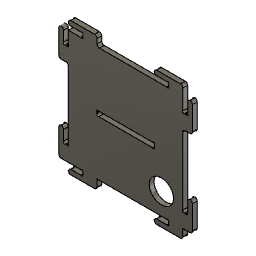
Side_HeatGun_Cut1 (Autodesk Fusion 360 design; units mm, degrees)
Autodesk Fusion 360 part; units mm, degrees
sketch "Sketch1" plane through (0, 0, 0) normal (0, 0, 1) x (1, 0, 0)
  line L0 (0, 0) -> (304.8, 0)
  line L1 (304.8, 0) -> (304.8, -304.8)
  line L2 (304.8, -304.8) -> (0, -304.8)
  line L3 (0, -304.8) -> (0, 0)
  line L4 (304.8, 0) -> (304.8, 25.4)
  line L5 (304.8, -304.8) -> (304.8, -330.2)
  line L6 (0, 0) -> (76.2, 0) construction
  line L7 (0, -304.8) -> (76.2, -304.8) construction
  line L8 (76.2, -304.8) -> (76.2, -330.2)
  line L9 (304.8, -330.2) -> (228.6, -330.2)
  line L10 (76.2, -330.2) -> (0, -330.2)
  line L11 (0, -330.2) -> (0, -317.5)
  line L12 (0, -317.5) -> (38.1, -317.5)
  line L13 (38.1, -317.5) -> (38.1, -304.8)
  line L14 (228.6, -330.2) -> (228.6, -317.5)
  line L15 (228.6, -317.5) -> (266.7, -317.5)
  line L16 (266.7, -317.5) -> (266.7, -304.8)
  line L17 (304.8, 25.4) -> (228.6, 25.4)
  line L18 (228.6, 25.4) -> (228.6, 12.7)
  line L19 (228.6, 12.7) -> (266.7, 12.7)
  line L20 (266.7, 12.7) -> (266.7, 0)
  line L21 (76.2, 0) -> (76.2, 25.4)
  line L22 (76.2, 25.4) -> (0, 25.4)
  line L23 (0, 25.4) -> (0, 12.7)
  line L24 (0, 12.7) -> (38.1, 12.7)
  line L25 (38.1, 12.7) -> (38.1, 0)
  line L26 (152.4, 0) -> (152.4, -152.4) construction
  line L27 (228.6, -158.75) -> (76.2, -158.75)
  line L28 (76.2, -158.75) -> (76.2, -146.05)
  line L29 (76.2, -146.05) -> (228.6, -146.05)
  line L30 (228.6, -146.05) -> (228.6, -158.75)
  line L31 (228.6, -158.75) -> (76.2, -146.05) construction
  line L32 (76.2, -158.75) -> (228.6, -146.05) construction
  line L33 (0, 0) -> (0, -76.2) construction
  line L34 (0, -76.2) -> (-25.4, -76.2)
  line L35 (-25.4, -76.2) -> (-25.4, 0)
  line L36 (-25.4, 0) -> (-12.7, 0)
  line L37 (-12.7, 0) -> (-12.7, -38.1)
  line L38 (-12.7, -38.1) -> (0, -38.1)
  line L39 (0, -304.8) -> (-25.4, -304.8)
  line L40 (-25.4, -304.8) -> (-25.4, -228.6)
  line L41 (-25.4, -228.6) -> (-12.7, -228.6)
  line L42 (-12.7, -228.6) -> (-12.7, -266.7)
  line L43 (-12.7, -266.7) -> (0, -266.7)
  line L44 (304.8, -304.8) -> (330.2, -304.8)
  line L45 (330.2, -304.8) -> (330.2, -228.6)
  line L46 (330.2, -228.6) -> (317.5, -228.6)
  line L47 (317.5, -228.6) -> (317.5, -266.7)
  line L48 (317.5, -266.7) -> (304.8, -266.7)
  line L49 (304.8, 0) -> (304.8, -76.2) construction
  line L50 (304.8, -76.2) -> (330.2, -76.2)
  line L51 (330.2, -76.2) -> (330.2, 0)
  line L52 (330.2, 0) -> (317.5, 0)
  line L53 (317.5, 0) -> (317.5, -38.1)
  line L54 (317.5, -38.1) -> (304.8, -38.1)
  point P0 (152.4, -152.4)
  dimension "d1" = 304.8
  dimension "d2" = 304.8
  dimension "d3" = 25.4
  dimension "d4" = 25.4
  dimension "d5" = 76.2
  dimension "d6" = 76.2
  dimension "d7" = 25.4
  dimension "d8" = 76.2
  dimension "d9" = 12.7
  dimension "d10" = 76.2
  dimension "d11" = 38.1
  dimension "d12" = 25.4
  dimension "d13" = 38.1
  dimension "d14" = 152.4
  dimension "d15" = 152.4
  dimension "d16" = 12.7
  dimension "d17" = 76.2
  dimension "d18" = 25.4
  dimension "d19" = 76.2
  dimension "d20" = 12.7
  dimension "d21" = 38.1
  dimension "d22" = 76.2
  dimension "d23" = 38.1
  dimension "d24" = 76.2
  constraint horizontal L0
  constraint vertical L1
  constraint horizontal L2
  constraint vertical L3
  constraint coincident L0.start L3.end
  constraint perpendicular L0 L4
  constraint perpendicular L2 L5
  constraint perpendicular L3 L6
  constraint perpendicular L3 L7
  constraint perpendicular L2 L8
  constraint perpendicular L5 L9
  constraint perpendicular L8 L10
  constraint perpendicular L10 L11
  constraint perpendicular L11 L12
  constraint midpoint L7 L13.end
  constraint perpendicular L9 L14
  constraint perpendicular L14 L15
  constraint coincident L2 L16.end
  constraint perpendicular L2 L16
  constraint perpendicular L4 L17
  constraint perpendicular L17 L18
  constraint perpendicular L4 L19
  constraint coincident L0 L20.end
  constraint perpendicular L0 L20
  constraint perpendicular L0 L21
  constraint perpendicular L21 L22
  constraint perpendicular L22 L23
  constraint perpendicular L21 L24
  constraint midpoint L6 L25.end
  constraint perpendicular L6 L25
  constraint midpoint L0 L26.start
  constraint perpendicular L2 L26
  constraint horizontal L27
  constraint perpendicular L27 L28
  constraint parallel L27 L29
  constraint parallel L28 L30
  constraint coincident L31 P0
  constraint coincident L32 P0
  constraint coincident P0 L26.end
  constraint perpendicular L0 L33
  constraint perpendicular L3 L34
  constraint perpendicular L34 L35
  constraint perpendicular L35 L36
  constraint perpendicular L36 L37
  constraint midpoint L33 L38.end
  constraint perpendicular L3 L39
  constraint perpendicular L39 L40
  constraint perpendicular L40 L41
  constraint perpendicular L41 L42
  constraint coincident L3 L43.end
  constraint perpendicular L3 L43
  constraint perpendicular L5 L44
  constraint perpendicular L2 L45
  constraint perpendicular L5 L46
  constraint perpendicular L46 L47
  constraint coincident L1 L48.end
  constraint perpendicular L1 L48
  constraint perpendicular L0 L49
  constraint perpendicular L1 L50
  constraint perpendicular L50 L51
  constraint perpendicular L1 L52
  constraint perpendicular L50 L53
  constraint midpoint L49 L54.end
  constraint perpendicular L49 L54
  measures "d1" distance of L0.start L0.end
  measures "d2" distance of L0.start L2.end
  measures "d3" distance of L0.end L4.end
  measures "d4" distance of L1.end L5.end
  measures "d5" distance of L0.start L6.end
  measures "d6" distance of L2.end L7.end
  measures "d7" distance of L7.end L8.end
  measures "d8" distance of L5.end L9.end
  measures "d9" distance of L9.end L14.end
  measures "d10" distance of L4.end L17.end
  measures "d11" distance of L18.end L19.end
  measures "d12" distance of L6.end L21.end
  measures "d13" distance of L23.end L24.end
  measures "d14" distance of L26.start P0
  measures "d15" distance of L28.end L29.end
  measures "d16" distance of L27.end L28.end
  measures "d17" distance of L0.start L33.end
  measures "d18" distance of L33.end L34.end
  measures "d19" distance of L34.end L35.end
  measures "d20" distance of L35.end L36.end
  measures "d21" distance of L36.end L37.end
  measures "d22" distance of L39.end L40.end
  measures "d23" distance of L41.end L42.end
  measures "d24" distance of L0.end L49.end
extrude "Extrude1" add sketch "Sketch1" along normal blind 12.7 makes body 1
fillet "Fillet1" radius 6.35 27 edges at (-25.4, 0, 6.35) (-12.7, 0, 6.35) (-25.4, -76.2, 6.35) (0, -76.2, 6.35) (0, 25.4, 6.35) (0, 12.7, 6.35) (76.2, 25.4, 6.35) (76.2, 0, 6.35) (228.6, 25.4, 6.35) (228.6, 12.7, 6.35) (304.8, 25.4, 6.35) (317.5, 0, 6.35) (330.2, 0, 6.35) (330.2, -76.2, 6.35) (304.8, -76.2, 6.35) (330.2, -228.6, 6.35) (317.5, -228.6, 6.35) (330.2, -304.8, 6.35) (304.8, -330.2, 6.35) (228.6, -317.5, 6.35) (228.6, -330.2, 6.35) (0, -317.5, 6.35) (0, -330.2, 6.35) (76.2, -330.2, 6.35) (-25.4, -304.8, 6.35) (-25.4, -228.6, 6.35) (-12.7, -228.6, 6.35) on bodies 1
sketch "Sketch2" plane through (0, 0, 12.7) normal (0, 0, 1) x (1, 0, 0)
  arc A0 (-12.7, -234.95) -> (-19.05, -228.6) centre (-19.05, -234.95) ccw
  arc A1 (-19.05, -228.6) -> (-25.4, -234.95) centre (-19.05, -234.95) ccw
  line L0 (-25.4, -234.95) -> (-25.4, -298.45)
  arc A2 (-25.4, -298.45) -> (-19.05, -304.8) centre (-19.05, -298.45) ccw
  line L1 (-19.05, -304.8) -> (38.1, -304.8)
  line L2 (38.1, -304.8) -> (38.1, -317.5)
  line L3 (38.1, -317.5) -> (6.35, -317.5)
  arc A3 (6.35, -317.5) -> (0, -323.85) centre (6.35, -323.85) ccw
  arc A4 (0, -323.85) -> (6.35, -330.2) centre (6.35, -323.85) ccw
  line L4 (6.35, -330.2) -> (69.85, -330.2)
  arc A5 (69.85, -330.2) -> (76.2, -323.85) centre (69.85, -323.85) ccw
  line L5 (76.2, -323.85) -> (76.2, -304.8)
  line L6 (76.2, -304.8) -> (266.7, -304.8)
  line L7 (266.7, -304.8) -> (266.7, -317.5)
  line L8 (266.7, -317.5) -> (234.95, -317.5)
  arc A6 (234.95, -317.5) -> (234.95, -330.2) centre (234.95, -323.85) ccw
  line L9 (234.95, -330.2) -> (298.45, -330.2)
  arc A7 (298.45, -330.2) -> (304.8, -323.85) centre (298.45, -323.85) ccw
  line L10 (304.8, -323.85) -> (304.8, -304.8)
  line L11 (304.8, -304.8) -> (323.85, -304.8)
  arc A8 (323.85, -304.8) -> (330.2, -298.45) centre (323.85, -298.45) ccw
  line L12 (330.2, -298.45) -> (330.2, -234.95)
  arc A9 (330.2, -234.95) -> (323.85, -228.6) centre (323.85, -234.95) ccw
  arc A10 (323.85, -228.6) -> (317.5, -234.95) centre (323.85, -234.95) ccw
  line L13 (317.5, -234.95) -> (317.5, -266.7)
  line L14 (317.5, -266.7) -> (304.8, -266.7)
  line L15 (304.8, -266.7) -> (304.8, -82.55)
  arc A11 (311.15, -76.2) -> (304.8, -82.55) centre (311.15, -82.55) ccw
  line L16 (311.15, -76.2) -> (323.85, -76.2)
  arc A12 (323.85, -76.2) -> (330.2, -69.85) centre (323.85, -69.85) ccw
  line L17 (330.2, -69.85) -> (330.2, -6.35)
  arc A13 (330.2, -6.35) -> (323.85, 0) centre (323.85, -6.35) ccw
  arc A14 (323.85, 0) -> (317.5, -6.35) centre (323.85, -6.35) ccw
  line L18 (317.5, -6.35) -> (317.5, -38.1)
  line L19 (317.5, -38.1) -> (304.8, -38.1)
  line L20 (304.8, -38.1) -> (304.8, 19.05)
  arc A15 (304.8, 19.05) -> (298.45, 25.4) centre (298.45, 19.05) ccw
  line L21 (298.45, 25.4) -> (234.95, 25.4)
  arc A16 (234.95, 25.4) -> (228.6, 19.05) centre (234.95, 19.05) ccw
  arc A17 (228.6, 19.05) -> (234.95, 12.7) centre (234.95, 19.05) ccw
  line L22 (234.95, 12.7) -> (266.7, 12.7)
  line L23 (266.7, 12.7) -> (266.7, 0)
  line L24 (266.7, 0) -> (82.55, 0)
  arc A18 (76.2, 6.35) -> (82.55, 0) centre (82.55, 6.35) ccw
  line L25 (76.2, 6.35) -> (76.2, 19.05)
  arc A19 (76.2, 19.05) -> (69.85, 25.4) centre (69.85, 19.05) ccw
  line L26 (69.85, 25.4) -> (6.35, 25.4)
  arc A20 (6.35, 25.4) -> (6.35, 12.7) centre (6.35, 19.05) ccw
  line L27 (6.35, 12.7) -> (38.1, 12.7)
  line L28 (38.1, 12.7) -> (38.1, 0)
  line L29 (38.1, 0) -> (0, 0)
  line L30 (0, 0) -> (0, -38.1)
  line L31 (0, -38.1) -> (-12.7, -38.1)
  line L32 (-12.7, -38.1) -> (-12.7, -6.35)
  arc A21 (-12.7, -6.35) -> (-25.4, -6.35) centre (-19.05, -6.35) ccw
  line L33 (-25.4, -6.35) -> (-25.4, -69.85)
  arc A22 (-25.4, -69.85) -> (-19.05, -76.2) centre (-19.05, -69.85) ccw
  line L34 (-19.05, -76.2) -> (-6.35, -76.2)
  arc A23 (0, -82.55) -> (-6.35, -76.2) centre (-6.35, -82.55) ccw
  line L35 (0, -82.55) -> (0, -266.7)
  line L36 (0, -266.7) -> (-12.7, -266.7)
  line L37 (-12.7, -266.7) -> (-12.7, -234.95)
  line L38 (76.2, -146.05) -> (228.6, -146.05)
  line L39 (228.6, -146.05) -> (228.6, -158.75)
  line L40 (228.6, -158.75) -> (76.2, -158.75)
  line L41 (76.2, -158.75) -> (76.2, -146.05)
copy_body "Body->Comp1" bodies 1 removing the originals makes body 2 in component "Component"
sketch "Sketch3" plane through (0, 0, 12.7) normal (0, 0, 1) x (1, 0, 0)
  arc A0 (-12.7, -234.95) -> (-19.05, -228.6) centre (-19.05, -234.95) ccw
  arc A1 (-19.05, -228.6) -> (-25.4, -234.95) centre (-19.05, -234.95) ccw
  line L0 (-25.4, -234.95) -> (-25.4, -298.45)
  arc A2 (-25.4, -298.45) -> (-19.05, -304.8) centre (-19.05, -298.45) ccw
  line L1 (-19.05, -304.8) -> (38.1, -304.8)
  line L2 (38.1, -304.8) -> (38.1, -317.5)
  line L3 (38.1, -317.5) -> (6.35, -317.5)
  arc A3 (6.35, -317.5) -> (0, -323.85) centre (6.35, -323.85) ccw
  arc A4 (0, -323.85) -> (6.35, -330.2) centre (6.35, -323.85) ccw
  line L4 (6.35, -330.2) -> (69.85, -330.2)
  arc A5 (69.85, -330.2) -> (76.2, -323.85) centre (69.85, -323.85) ccw
  line L5 (76.2, -323.85) -> (76.2, -304.8)
  line L6 (76.2, -304.8) -> (266.7, -304.8)
  line L7 (266.7, -304.8) -> (266.7, -317.5)
  line L8 (266.7, -317.5) -> (234.95, -317.5)
  arc A6 (234.95, -317.5) -> (234.95, -330.2) centre (234.95, -323.85) ccw
  line L9 (234.95, -330.2) -> (298.45, -330.2)
  arc A7 (298.45, -330.2) -> (304.8, -323.85) centre (298.45, -323.85) ccw
  line L10 (304.8, -323.85) -> (304.8, -304.8)
  line L11 (304.8, -304.8) -> (323.85, -304.8)
  arc A8 (323.85, -304.8) -> (330.2, -298.45) centre (323.85, -298.45) ccw
  line L12 (330.2, -298.45) -> (330.2, -234.95)
  arc A9 (330.2, -234.95) -> (323.85, -228.6) centre (323.85, -234.95) ccw
  arc A10 (323.85, -228.6) -> (317.5, -234.95) centre (323.85, -234.95) ccw
  line L13 (317.5, -234.95) -> (317.5, -266.7)
  line L14 (317.5, -266.7) -> (304.8, -266.7)
  line L15 (304.8, -266.7) -> (304.8, -82.55)
  arc A11 (311.15, -76.2) -> (304.8, -82.55) centre (311.15, -82.55) ccw
  line L16 (311.15, -76.2) -> (323.85, -76.2)
  arc A12 (323.85, -76.2) -> (330.2, -69.85) centre (323.85, -69.85) ccw
  line L17 (330.2, -69.85) -> (330.2, -6.35)
  arc A13 (330.2, -6.35) -> (323.85, 0) centre (323.85, -6.35) ccw
  arc A14 (323.85, 0) -> (317.5, -6.35) centre (323.85, -6.35) ccw
  line L18 (317.5, -6.35) -> (317.5, -38.1)
  line L19 (317.5, -38.1) -> (304.8, -38.1)
  line L20 (304.8, -38.1) -> (304.8, 19.05)
  arc A15 (304.8, 19.05) -> (298.45, 25.4) centre (298.45, 19.05) ccw
  line L21 (298.45, 25.4) -> (234.95, 25.4)
  arc A16 (234.95, 25.4) -> (228.6, 19.05) centre (234.95, 19.05) ccw
  arc A17 (228.6, 19.05) -> (234.95, 12.7) centre (234.95, 19.05) ccw
  line L22 (234.95, 12.7) -> (266.7, 12.7)
  line L23 (266.7, 12.7) -> (266.7, 0)
  line L24 (266.7, 0) -> (82.55, 0)
  arc A18 (76.2, 6.35) -> (82.55, 0) centre (82.55, 6.35) ccw
  line L25 (76.2, 6.35) -> (76.2, 19.05)
  arc A19 (76.2, 19.05) -> (69.85, 25.4) centre (69.85, 19.05) ccw
  line L26 (69.85, 25.4) -> (6.35, 25.4)
  arc A20 (6.35, 25.4) -> (6.35, 12.7) centre (6.35, 19.05) ccw
  line L27 (6.35, 12.7) -> (38.1, 12.7)
  line L28 (38.1, 12.7) -> (38.1, 0)
  line L29 (38.1, 0) -> (0, 0)
  line L30 (0, 0) -> (0, -38.1)
  line L31 (0, -38.1) -> (-12.7, -38.1)
  line L32 (-12.7, -38.1) -> (-12.7, -6.35)
  arc A21 (-12.7, -6.35) -> (-25.4, -6.35) centre (-19.05, -6.35) ccw
  line L33 (-25.4, -6.35) -> (-25.4, -69.85)
  arc A22 (-25.4, -69.85) -> (-19.05, -76.2) centre (-19.05, -69.85) ccw
  line L34 (-19.05, -76.2) -> (-6.35, -76.2)
  arc A23 (0, -82.55) -> (-6.35, -76.2) centre (-6.35, -82.55) ccw
  line L35 (0, -82.55) -> (0, -266.7)
  line L36 (0, -266.7) -> (-12.7, -266.7)
  line L37 (-12.7, -266.7) -> (-12.7, -234.95)
  line L38 (76.2, -146.05) -> (228.6, -146.05)
  line L39 (228.6, -146.05) -> (228.6, -158.75)
  line L40 (228.6, -158.75) -> (76.2, -158.75)
  line L41 (76.2, -158.75) -> (76.2, -146.05)
  line L42 (304.8, -304.8) -> (247.65, -304.8) construction
  line L43 (247.65, -304.8) -> (247.65, -247.65) construction
  ellipse E0 centre (247.65, -247.65) end of major axis (247.65, -216.535) minor radius 32.385
  line L44 (247.65, -278.765) -> (247.65, -216.535)
  line L45 (280.035, -247.65) -> (215.265, -247.65)
  dimension "d29" = 57.15
  dimension "d30" = 57.15
  dimension "d32" = 62.23
  dimension "d33" = 64.77
  constraint coincident L10.end L11.start
  constraint perpendicular L7 L42
  constraint perpendicular L6 L43
  constraint coincident L43.end E0.centre
  constraint parallel L43 L44
  constraint coincident E0 L44.start
  constraint coincident E0 L44.end
  constraint coincident E0 L45.start
  constraint coincident E0 L45.end
  measures "d29" distance of L10.end L42.end
  measures "d30" distance of L42.end L43.end
  measures "d32" distance of E0
extrude "Extrude1'" cut sketch "Sketch3" against normal up to surface (12.7 mm away) contours E0 L44 L45 | E0 L44 L45 | E0 L44 L45 | E0 L44 L45 bodies 2 in component "Component"
ref_plane "WorkPlane1" through (38.1, 12.7, 0) normal (0, 0, 1) x (1, 0, 0)
sketch "Sketch4" plane through (38.1, 12.7, 0) normal (0, 0, 1) x (1, 0, 0)
  line L0 (-31.75, 0) -> (0, 0) construction
  line L1 (0, 0) -> (0, -12.7) construction
  line L2 (0, 0) -> (-2.2451, -2.2451) construction
  circle A0 centre (-2.2451, -2.2451) radius 3.175
  dimension "d37" = 3.175
  constraint coincident L0.end L1.start
  constraint coincident L0.end A0
  measures "d37" distance of L0.end L2.end
sweep "Sweep1" cut kept parallel profiles "Sketch4" along 1 edges at (38.1, 12.7, 6.35) section 1 on bodies 2 bodies 2 in component "Component"
ref_plane "WorkPlane2" through (38.1, 0, 0) normal (0, 0, 1) x (1, 0, 0)
sketch "Sketch5" plane through (38.1, 0, 0) normal (0, 0, 1) x (1, 0, 0)
  line L0 (0, 8.2099) -> (0, 0) construction
  line L1 (-38.1, 0) -> (0, 0) construction
  line L2 (0, 0) -> (-2.2451, 2.2451) construction
  circle A0 centre (-2.2451, 2.2451) radius 3.175
  dimension "d45" = 3.175
  constraint coincident L0.end L1.end
  constraint coincident L0.end A0
  measures "d45" distance of L0.end L2.end
sweep "Sweep2" cut kept parallel profiles "Sketch5" along 1 edges at (38.1, 0, 6.35) section 1 on bodies 2 bodies 2 in component "Component"
ref_plane "WorkPlane3" through (0, -38.1, 0) normal (0, 0, 1) x (1, 0, 0)
sketch "Sketch6" plane through (0, -38.1, 0) normal (0, 0, 1) x (1, 0, 0)
  line L0 (0, 0) -> (0, 38.1) construction
  line L1 (-12.7, 0) -> (0, 0) construction
  line L2 (0, 0) -> (-2.2451, 2.2451) construction
  circle A0 centre (-2.2451, 2.2451) radius 3.175
  dimension "d53" = 3.175
  constraint coincident L0.start L1.end
  constraint coincident L0.start A0
  measures "d53" distance of L0.start L2.end
sweep "Sweep3" cut kept parallel profiles "Sketch6" along 1 edges at (0, -38.1, 6.35) section 1 on bodies 2 bodies 2 in component "Component"
ref_plane "WorkPlane4" through (-12.7, -38.1, 0) normal (0, 0, 1) x (1, 0, 0)
sketch "Sketch7" plane through (-12.7, -38.1, 0) normal (0, 0, 1) x (1, 0, 0)
  line L0 (0, 0) -> (8.2099, 0) construction
  line L1 (0, 31.75) -> (0, 0) construction
  line L2 (0, 0) -> (2.2451, 2.2451) construction
  circle A0 centre (2.2451, 2.2451) radius 3.175
  dimension "d61" = 3.175
  constraint coincident L0.start L1.end
  constraint coincident L0.start A0
  measures "d61" distance of L0.start L2.end
sweep "Sweep4" cut kept parallel profiles "Sketch7" along 1 edges at (-12.7, -38.1, 6.35) section 1 on bodies 2 bodies 2 in component "Component"
ref_plane "WorkPlane5" through (304.8, -38.1, 0) normal (0, 0, 1) x (1, 0, 0)
sketch "Sketch8" plane through (304.8, -38.1, 0) normal (0, 0, 1) x (1, 0, 0)
  line L0 (12.7, 0) -> (0, 0) construction
  line L1 (0, 57.15) -> (0, 0) construction
  line L2 (0, 0) -> (2.2451, 2.2451) construction
  circle A0 centre (2.2451, 2.2451) radius 3.175
  dimension "d69" = 3.175
  constraint coincident L0.end L1.end
  constraint coincident L0.end A0
  measures "d69" distance of L0.end L2.end
sweep "Sweep5" cut kept parallel profiles "Sketch8" along 1 edges at (304.8, -38.1, 6.35) section 1 on bodies 2 bodies 2 in component "Component"
ref_plane "WorkPlane6" through (317.5, -38.1, 0) normal (0, 0, 1) x (1, 0, 0)
sketch "Sketch9" plane through (317.5, -38.1, 0) normal (0, 0, 1) x (1, 0, 0)
  line L0 (0, 31.75) -> (0, 0) construction
  line L1 (0, 0) -> (-8.2099, 0) construction
  line L2 (0, 0) -> (-2.2451, 2.2451) construction
  circle A0 centre (-2.2451, 2.2451) radius 3.175
  dimension "d77" = 3.175
  constraint coincident L0.end L1.start
  constraint coincident L0.end A0
  measures "d77" distance of L0.end L2.end
sweep "Sweep6" cut kept parallel profiles "Sketch9" along 1 edges at (317.5, -38.1, 6.35) section 1 on bodies 2 bodies 2 in component "Component"
ref_plane "WorkPlane7" through (266.7, 12.7, 0) normal (0, 0, 1) x (1, 0, 0)
sketch "Sketch10" plane through (266.7, 12.7, 0) normal (0, 0, 1) x (1, 0, 0)
  line L0 (-31.75, 0) -> (0, 0) construction
  line L1 (0, 0) -> (0, -12.7) construction
  line L2 (0, 0) -> (-2.2451, -2.2451) construction
  circle A0 centre (-2.2451, -2.2451) radius 3.175
  dimension "d85" = 3.175
  constraint coincident L0.end L1.start
  constraint coincident L0.end A0
  measures "d85" distance of L0.end L2.end
sweep "Sweep7" cut kept parallel profiles "Sketch10" along 1 edges at (266.7, 12.7, 6.35) section 1 on bodies 2 bodies 2 in component "Component"
ref_plane "WorkPlane8" through (266.7, 0, 0) normal (0, 0, 1) x (1, 0, 0)
sketch "Sketch11" plane through (266.7, 0, 0) normal (0, 0, 1) x (1, 0, 0)
  line L0 (0, 8.2099) -> (0, 0) construction
  line L1 (-184.15, 0) -> (0, 0) construction
  line L2 (0, 0) -> (-2.2451, 2.2451) construction
  circle A0 centre (-2.2451, 2.2451) radius 3.175
  dimension "d93" = 3.175
  constraint coincident L0.end L1.end
  constraint coincident L0.end A0
  measures "d93" distance of L0.end L2.end
sweep "Sweep8" cut kept parallel profiles "Sketch11" along 1 edges at (266.7, 0, 6.35) section 1 on bodies 2 bodies 2 in component "Component"
ref_plane "WorkPlane9" through (317.5, -266.7, 0) normal (0, 0, 1) x (1, 0, 0)
sketch "Sketch12" plane through (317.5, -266.7, 0) normal (0, 0, 1) x (1, 0, 0)
  line L0 (0, 31.75) -> (0, 0) construction
  line L1 (0, 0) -> (-12.7, 0) construction
  line L2 (0, 0) -> (-2.2451, 2.2451) construction
  circle A0 centre (-2.2451, 2.2451) radius 3.175
  dimension "d101" = 3.175
  constraint coincident L0.end L1.start
  constraint coincident L0.end A0
  measures "d101" distance of L0.end L2.end
sweep "Sweep9" cut kept parallel profiles "Sketch12" along 1 edges at (317.5, -266.7, 6.35) section 1 on bodies 2 bodies 2 in component "Component"
ref_plane "WorkPlane10" through (304.8, -266.7, 0) normal (0, 0, 1) x (1, 0, 0)
sketch "Sketch13" plane through (304.8, -266.7, 0) normal (0, 0, 1) x (1, 0, 0)
  line L0 (8.2099, 0) -> (0, 0) construction
  line L1 (0, 184.15) -> (0, 0) construction
  line L2 (0, 0) -> (2.2451, 2.2451) construction
  circle A0 centre (2.2451, 2.2451) radius 3.175
  dimension "d109" = 3.175
  constraint coincident L0.end L1.end
  constraint coincident L0.end A0
  measures "d109" distance of L0.end L2.end
sweep "Sweep10" cut kept parallel profiles "Sketch13" along 1 edges at (304.8, -266.7, 6.35) section 1 on bodies 2 bodies 2 in component "Component"
ref_plane "WorkPlane11" through (266.7, -304.8, 0) normal (0, 0, 1) x (1, 0, 0)
sketch "Sketch14" plane through (266.7, -304.8, 0) normal (0, 0, 1) x (1, 0, 0)
  line L0 (0, 0) -> (-190.5, 0) construction
  line L1 (0, -12.7) -> (0, 0) construction
  line L2 (0, 0) -> (-2.2451, -2.2451) construction
  circle A0 centre (-2.2451, -2.2451) radius 3.175
  dimension "d117" = 3.175
  constraint coincident L0.start L1.end
  constraint coincident L0.start A0
  measures "d117" distance of L0.start L2.end
sweep "Sweep11" cut kept parallel profiles "Sketch14" along 1 edges at (266.7, -304.8, 6.35) section 1 on bodies 2 bodies 2 in component "Component"
ref_plane "WorkPlane12" through (266.7, -317.5, 0) normal (0, 0, 1) x (1, 0, 0)
sketch "Sketch15" plane through (266.7, -317.5, 0) normal (0, 0, 1) x (1, 0, 0)
  line L0 (0, 0) -> (0, 8.2099) construction
  line L1 (-31.75, 0) -> (0, 0) construction
  line L2 (0, 0) -> (-2.2451, 2.2451) construction
  circle A0 centre (-2.2451, 2.2451) radius 3.175
  dimension "d125" = 3.175
  constraint coincident L0.start L1.end
  constraint coincident L0.start A0
  measures "d125" distance of L0.start L2.end
sweep "Sweep12" cut kept parallel profiles "Sketch15" along 1 edges at (266.7, -317.5, 6.35) section 1 on bodies 2 bodies 2 in component "Component"
ref_plane "WorkPlane13" through (228.6, -158.75, 0) normal (0, 0, 1) x (1, 0, 0)
sketch "Sketch16" plane through (228.6, -158.75, 0) normal (0, 0, 1) x (1, 0, 0)
  line L0 (0, 12.7) -> (0, 0) construction
  line L1 (0, 0) -> (-152.4, 0) construction
  line L2 (0, 0) -> (-2.2451, 2.2451) construction
  circle A0 centre (-2.2451, 2.2451) radius 3.175
  dimension "d133" = 3.175
  constraint coincident L0.end L1.start
  constraint coincident L0.end A0
  measures "d133" distance of L0.end L2.end
sweep "Sweep13" cut kept parallel profiles "Sketch16" along 1 edges at (228.6, -158.75, 6.35) section 1 on bodies 2 bodies 2 in component "Component"
ref_plane "WorkPlane14" through (76.2, -158.75, 0) normal (0, 0, 1) x (1, 0, 0)
sketch "Sketch17" plane through (76.2, -158.75, 0) normal (0, 0, 1) x (1, 0, 0)
  line L0 (147.9099, 0) -> (0, 0) construction
  line L1 (0, 0) -> (0, 12.7) construction
  line L2 (0, 0) -> (2.2451, 2.2451) construction
  circle A0 centre (2.2451, 2.2451) radius 3.175
  dimension "d141" = 3.175
  constraint coincident L0.end L1.start
  constraint coincident L0.end A0
  measures "d141" distance of L0.end L2.end
sweep "Sweep14" cut kept parallel profiles "Sketch17" along 1 edges at (76.2, -158.75, 6.35) section 1 on bodies 2 bodies 2 in component "Component"
ref_plane "WorkPlane15" through (76.2, -146.05, 0) normal (0, 0, 1) x (1, 0, 0)
sketch "Sketch18" plane through (76.2, -146.05, 0) normal (0, 0, 1) x (1, 0, 0)
  line L0 (0, 0) -> (152.4, 0) construction
  line L1 (0, -8.2099) -> (0, 0) construction
  line L2 (0, 0) -> (2.2451, -2.2451) construction
  circle A0 centre (2.2451, -2.2451) radius 3.175
  dimension "d149" = 3.175
  constraint coincident L0.start L1.end
  constraint coincident L0.start A0
  measures "d149" distance of L0.start L2.end
sweep "Sweep15" cut kept parallel profiles "Sketch18" along 1 edges at (76.2, -146.05, 6.35) section 1 on bodies 2 bodies 2 in component "Component"
ref_plane "WorkPlane16" through (228.6, -146.05, 0) normal (0, 0, 1) x (1, 0, 0)
sketch "Sketch19" plane through (228.6, -146.05, 0) normal (0, 0, 1) x (1, 0, 0)
  line L0 (-147.9099, 0) -> (0, 0) construction
  line L1 (0, 0) -> (0, -8.2099) construction
  line L2 (0, 0) -> (-2.2451, -2.2451) construction
  circle A0 centre (-2.2451, -2.2451) radius 3.175
  dimension "d157" = 3.175
  constraint coincident L0.end L1.start
  constraint coincident L0.end A0
  measures "d157" distance of L0.end L2.end
sweep "Sweep16" cut kept parallel profiles "Sketch19" along 1 edges at (228.6, -146.05, 6.35) section 1 on bodies 2 bodies 2 in component "Component"
ref_plane "WorkPlane17" through (38.1, -304.8, 0) normal (0, 0, 1) x (1, 0, 0)
sketch "Sketch20" plane through (38.1, -304.8, 0) normal (0, 0, 1) x (1, 0, 0)
  line L0 (0, 0) -> (-57.15, 0) construction
  line L1 (0, -12.7) -> (0, 0) construction
  line L2 (0, 0) -> (-2.2451, -2.2451) construction
  circle A0 centre (-2.2451, -2.2451) radius 3.175
  dimension "d165" = 3.175
  constraint coincident L0.start L1.end
  constraint coincident L0.start A0
  measures "d165" distance of L0.start L2.end
sweep "Sweep17" cut kept parallel profiles "Sketch20" along 1 edges at (38.1, -304.8, 6.35) section 1 on bodies 2 bodies 2 in component "Component"
ref_plane "WorkPlane18" through (38.1, -317.5, 0) normal (0, 0, 1) x (1, 0, 0)
sketch "Sketch21" plane through (38.1, -317.5, 0) normal (0, 0, 1) x (1, 0, 0)
  line L0 (0, 0) -> (0, 8.2099) construction
  line L1 (-31.75, 0) -> (0, 0) construction
  line L2 (0, 0) -> (-2.2451, 2.2451) construction
  circle A0 centre (-2.2451, 2.2451) radius 3.175
  dimension "d173" = 3.175
  constraint coincident L0.start L1.end
  constraint coincident L0.start A0
  measures "d173" distance of L0.start L2.end
sweep "Sweep18" cut kept parallel profiles "Sketch21" along 1 edges at (38.1, -317.5, 6.35) section 1 on bodies 2 bodies 2 in component "Component"
ref_plane "WorkPlane19" through (0, -266.7, 0) normal (0, 0, 1) x (1, 0, 0)
sketch "Sketch22" plane through (0, -266.7, 0) normal (0, 0, 1) x (1, 0, 0)
  line L0 (0, 0) -> (0, 184.15) construction
  line L1 (-12.7, 0) -> (0, 0) construction
  line L2 (0, 0) -> (-2.2451, 2.2451) construction
  circle A0 centre (-2.2451, 2.2451) radius 3.175
  dimension "d181" = 3.175
  constraint coincident L0.start L1.end
  constraint coincident L0.start A0
  measures "d181" distance of L0.start L2.end
sweep "Sweep19" cut kept parallel profiles "Sketch22" along 1 edges at (0, -266.7, 6.35) section 1 on bodies 2 bodies 2 in component "Component"
ref_plane "WorkPlane20" through (-12.7, -266.7, 0) normal (0, 0, 1) x (1, 0, 0)
sketch "Sketch23" plane through (-12.7, -266.7, 0) normal (0, 0, 1) x (1, 0, 0)
  line L0 (0, 0) -> (8.2099, 0) construction
  line L1 (0, 31.75) -> (0, 0) construction
  line L2 (0, 0) -> (2.2451, 2.2451) construction
  circle A0 centre (2.2451, 2.2451) radius 3.175
  dimension "d189" = 3.175
  constraint coincident L0.start L1.end
  constraint coincident L0.start A0
  measures "d189" distance of L0.start L2.end
sweep "Sweep20" cut kept parallel profiles "Sketch23" along 1 edges at (-12.7, -266.7, 6.35) section 1 on bodies 2 bodies 2 in component "Component"
component "Component" placed x (1, 0, 0) y (0, 1, 0) z (0, 0, 1) at (0, 0, 0)
equation "d32 = HeatGunEllipseHeight"
equation "d33 = HeatGunEllipseWidth"
equation "d37 = 0.25 in / 2 + 0.00 in"
equation "d45 = 0.25 in / 2 + 0.00 in"
equation "d53 = 0.25 in / 2 + 0.00 in"
equation "d61 = 0.25 in / 2 + 0.00 in"
equation "d69 = 0.25 in / 2 + 0.00 in"
equation "d77 = 0.25 in / 2 + 0.00 in"
equation "d85 = 0.25 in / 2 + 0.00 in"
equation "d93 = 0.25 in / 2 + 0.00 in"
equation "d101 = 0.25 in / 2 + 0.00 in"
equation "d109 = 0.25 in / 2 + 0.00 in"
equation "d117 = 0.25 in / 2 + 0.00 in"
equation "d125 = 0.25 in / 2 + 0.00 in"
equation "d133 = 0.25 in / 2 + 0.00 in"
equation "d141 = 0.25 in / 2 + 0.00 in"
equation "d149 = 0.25 in / 2 + 0.00 in"
equation "d157 = 0.25 in / 2 + 0.00 in"
equation "d165 = 0.25 in / 2 + 0.00 in"
equation "d173 = 0.25 in / 2 + 0.00 in"
equation "d181 = 0.25 in / 2 + 0.00 in"
equation "d189 = 0.25 in / 2 + 0.00 in"
equation "HeatGunEllipseWidth = 2.55 in"
equation "HeatGunEllipseHeight = 2.45 in"
